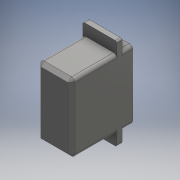
# Autodesk Inventor part: Servo
Saved by Autodesk Inventor 2016 (Build 200138000, 138)
## iProperties
Created: 2016-11-07
Part Number: Servo
Material: Generic
Document SubType Name: Modeling
Designer: Matt Cocca
Density: 1 g/cm^3
Appearance: Smooth - Medium Gray
Author: Matt Cocca
Autodesk Inventor part; units mm, degrees
ref_plane "YZ Plane" through (0, 0, 0) normal (1, 0, 0) x (0, 1, 0)
ref_plane "XZ Plane" through (0, 0, 0) normal (0, 1, 0) x (-1, 0, 0)
ref_plane "XY Plane" through (0, 0, 0) normal (0, 0, 1) x (1, 0, 0)
sketch "Sketch1" plane through (0, 0, 0) normal (0, 1, 0) x (-1, 0, 0)
  line L0 (0, 0) -> (-20, 0)
  line L1 (-20, 0) -> (-20, -40.3)
  line L2 (-20, -40.3) -> (0, -40.3)
  line L3 (0, -40.3) -> (0, 0)
  dimension "d0" = 20
  dimension "d1" = 40.3
  constraints: 8 end point, 2 parallel, 1 horizontal, 1 perpendicular
  measures "d0" distance of L2.end L1.end
  measures "d1" distance of L1.end L0.end
extrude "Extrusion1" add sketch "Sketch1" along normal blind 36.6
fillet "Fillet1" radius 2 4 edges at (20, 18.3, 0) (0, 18.3, 0) (20, 18.3, -40.3) (0, 18.3, -40.3)
chamfer "Chamfer1" distance 2 angle 45 8 edges at (20, 0, -20.15) (19.4142, 0, -39.7142) (10, 0, -40.3) (0.5858, 0, -39.7142) (0, 0, -20.15) (0.5858, 0, -0.5858) (10, 0, 0) (19.4142, 0, -0.5858)
fillet "Fillet2" radius 1 8 edges at (19.4142, 36.6, -39.7142) (10, 36.6, -40.3) (0.5858, 36.6, -39.7142) (0, 36.6, -20.15) (0.5858, 36.6, -0.5858) (10, 36.6, 0) (19.4142, 36.6, -0.5858) (20, 36.6, -20.15)
sketch "Sketch2" plane through (0, 36.6, 0) normal (0, 1, 0) x (1, 0, 0)
  line L0 (2, 0) -> (18, 0) projected
  line L1 (18, 0) -> (2, 0) projected
  line L2 (10, 0) -> (10, 33.5)
  line L3 (10, 0) -> (43.5, 0) construction
  circle A0 centre (10, 33.5) radius 3
  point P0 (0, 0)
  dimension "d9" = 33.5
  dimension "d10" = 90
  dimension "d11" = 6
  constraints: 4 end point, 1 centre point, 1 coincident, 1 horizontal, 1 midpoint, 1 perpendicular, 1 vertical
  measures "d9" distance of L2.start L2.end
  measures "d10" angle of L3 L2
  measures "d11" diameter of A0
extrude "Extrusion2" add sketch "Sketch2" along normal blind 5
sketch "Sketch3" plane through (2, 2, 0) normal (0, 0, 1) x (1, 0, 0)
  line L0 (0, -2) -> (16, -2) projected
  line L1 (18, 33.6) -> (18, 0) projected
  line L2 (-2, 27.6) -> (18, 27.6)
  line L3 (18, 27.6) -> (18, 24.6)
  line L4 (18, 24.6) -> (-2, 24.6)
  line L5 (-2, 24.6) -> (-2, 27.6)
  point P0 (-2, -2)
  dimension "d14" = 3
  dimension "d15" = 26.6
  constraints: 8 end point, 2 parallel, 1 horizontal, 1 perpendicular, 1 point on line
  measures "d14" distance of L2.end L3.end
  measures "d15" distance between parallel lines of L0 L4
extrude "Extrusion3" add sketch "Sketch3" along normal blind 6.65 and the other way blind 46.95
fillet "Fillet3" radius 1 4 edges at (20, 28.1, 6.65) (0, 28.1, 6.65) (20, 28.1, -46.95) (0, 28.1, -46.95)
body "Solid1"
